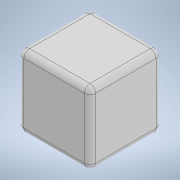
# Autodesk Inventor part: cube
Saved by Autodesk Inventor 2021 (Build 250183000, 183)
## iProperties
Created: 2020-06-12
Part Number: cube
Material: Generic
Document SubType Name: Modeling
Designer: dan
Density: 1 g/cm^3
Appearance: Default
Author: dan
Autodesk Inventor part; units mm, degrees
ref_plane "YZ Plane" through (0, 0, 0) normal (1, 0, 0) x (0, 1, 0)
ref_plane "XZ Plane" through (0, 0, 0) normal (0, 1, 0) x (-1, 0, 0)
ref_plane "XY Plane" through (0, 0, 0) normal (0, 0, 1) x (1, 0, 0)
sketch "Sketch1" plane through (0, 0, 0) normal (0, 0, 1) x (1, 0, 0)
  line L0 (-9.5, 9.5) -> (9.5, 9.5)
  line L1 (9.5, 9.5) -> (9.5, -9.5)
  line L2 (9.5, -9.5) -> (-9.5, -9.5)
  line L3 (-9.5, -9.5) -> (-9.5, 9.5)
  point P0 (0, 0)
  dimension "d0" = 19
  dimension "d1" = 19
  dimension "d2" = 9.5
  dimension "d3" = 9.5
  constraints: 8 end point, 2 parallel, 1 horizontal, 1 perpendicular
  measures "d0" distance of L0.start L0.end
  measures "d1" distance of L2.end L0.start
  measures "d2" distance from line of point (0, 0) L0
  measures "d3" distance from line of point (0, 0) L3
extrude "Extrusion1" add sketch "Sketch1" along normal blind 19
fillet "Fillet1" radius 1.5 12 edges at (9.5, 9.5, 9.5) (9.5, 0, 19) (9.5, 0, 0) (9.5, -9.5, 9.5) (-9.5, 9.5, 9.5) (-9.5, 0, 19) (-9.5, 0, 0) (-9.5, -9.5, 9.5) (0, -9.5, 19) (0, 9.5, 19) (0, 9.5, 0) (0, -9.5, 0)
body "Solid1"
